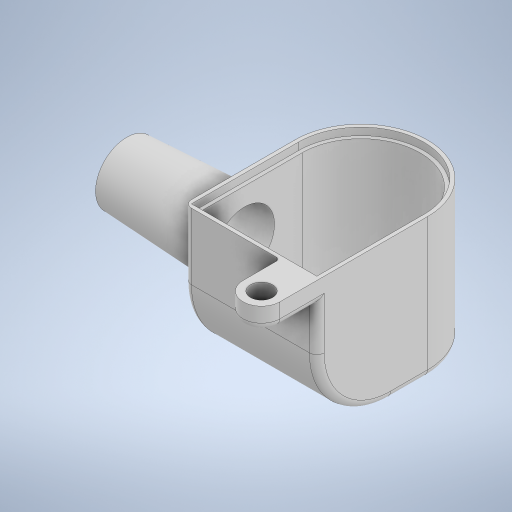
# Autodesk Inventor part: 薄殼1
Saved by Autodesk Inventor 2024.2 (Build 282272000, 272)
## iProperties
Created: 2024-03-28
Part Number: 薄殼1
Material: 一般
Document SubType Name: Modeling
Designer: User
Density: 1 g/cm^3
Appearance: 預設
Author: User
Autodesk Inventor part; units mm, degrees
ref_plane "YZ Plane" through (0, 0, 0) normal (1, 0, 0) x (0, 1, 0)
ref_plane "XZ Plane" through (0, 0, 0) normal (0, 1, 0) x (-1, 0, 0)
ref_plane "XY Plane" through (0, 0, 0) normal (0, 0, 1) x (1, 0, 0)
sketch "草圖2" plane through (0, 0, 0) normal (0, 1, 0) x (-1, 0, 0)
  line L0 (-0.3285, 0) -> (-18.3285, 0)
  line L1 (-18.3285, 0) -> (-18.3285, -15)
  line L2 (-0.3285, -15) -> (-0.3285, 0)
  arc A0 (-18.3285, -15) -> (-0.3285, -15) centre (-9.3285, -15) ccw
  point P0 (0, 0)
  dimension "d0" = 18
  dimension "d1" = 15
  constraints: 6 end point, 2 point on circle, 2 tangent, 1 centre point, 1 horizontal, 1 parallel, 1 perpendicular
  measures "d0" distance of L2.start L1.end
  measures "d1" distance of L1.end L0.end
extrude "擠出1" add sketch "草圖2" along normal blind 18
fillet "圓角1" radius 10 1 edges at (9.3285, 0, 0)
sketch "草圖3" plane through (0.3285, 0, -15) normal (-1, 0, 0) x (0, 0, 1)
  circle A0 centre (7.7956, 11.4963) radius 5
  point P0 (15, 0)
  dimension "d5" = 10
  constraints: 1 centre point
  measures "d5" diameter of A0
extrude "擠出2" add sketch "草圖3" along normal blind 15 draft -3
shell "薄殼1" thickness 1 removed faces 2 at (12.3285, 18, -5) at (-14.6715, 10.8436, -5.9606)
sketch "草圖5" plane through (0, 18, 0) normal (0, 1, 0) x (1, 0, 0)
  line L0 (18.3285, 15) -> (18.3285, 0)
  line L1 (18.3285, 0) -> (0.3285, 0)
  line L2 (0.3285, 0) -> (0.3285, 15)
  arc A0 (18.3285, 15) -> (0.3285, 15) centre (9.3285, 15) ccw
  line L3 (0.8285, 15) -> (0.8285, 0.5)
  line L4 (0.8285, 0.5) -> (17.8285, 0.5)
  line L5 (17.8285, 0.5) -> (17.8285, 15)
  arc A1 (17.8285, 15) -> (0.8285, 15) centre (9.3285, 15) ccw
  line L6 (0.3285, 15) -> (0.8285, 15)
  line L7 (17.8285, 15) -> (18.3285, 15)
  line L8 (0.8285, 0.5) -> (17.8285, 0.5)
  line L9 (18.3285, 0) -> (0.3285, 0)
  point P0 (0, 0)
  dimension "d10" = 0.5
  constraints: 20 end point, 4 equal length, 4 point on circle, 2 centre point, 2 horizontal, 2 tangent, 3 other
  measures "d10" radial gap between concentric circles of A0 A1
extrude "擠出3" add sketch "草圖5" along normal blind 1 contours L7 A1 L6 A0 | L0 L1 L2 L6 L3 L4 L5 L7
sketch "草圖6" plane through (0, 19, 0) normal (0, 1, 0) x (1, 0, 0)
  line L0 (18.3285, 0) -> (0.3285, 0) projected
  line L1 (18.3285, 0) -> (13.3285, 0)
  line L2 (13.3285, 0) -> (13.3285, -5)
  line L3 (18.3285, -5) -> (18.3285, 0)
  arc A0 (13.3285, -5) -> (18.3285, -5) centre (15.8285, -5) ccw
  circle A1 centre (15.8285, -5) radius 1.5
  point P0 (0, 0)
  dimension "d13" = 5
  dimension "d14" = 5
  constraints: 6 end point, 2 centre point, 2 point on circle, 1 coincident, 1 parallel, 1 perpendicular, 1 point on line
  measures "d13" distance of L0.start L1.end
  measures "d14" distance of L2.end L1.end
extrude "擠出4" add sketch "草圖6" against normal blind 3
fillet "圓角2" radius 0.5 1 edges at (13.3285, 17.5, 0)
fillet "圓角3" radius 1 11 edges at (0.3285, 0, -12.5) (9.3285, 0, -24) (18.3285, 0, -12.5) (18.3285, 2.9289, -2.9289) (18.3285, 13, 0) (0.3285, 14.5, 0) (0.3285, 2.9289, -2.9289) (13.3285, 16, 2.75) (13.182, 16, 0.1464) (18.3285, 16, 2.5) (15.8285, 16, 7.5)
